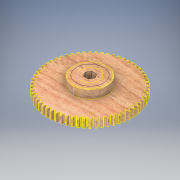
# Autodesk Inventor part: gear2
Saved by Autodesk Inventor 2018 (Build 220112000, 112)
## iProperties
Created: 2019-02-16
Part Number: gear2
Material: Generic
Description: SolidWorks IGES file using analytic representation for surfaces
Document SubType Name: Modeling
Designer: snipe
Density: 1 g/cm^3
Appearance: Default
Sending System: SolidWorks 2018
Preprocessor: SolidWorks 2018
Minimum Resolution: 0.0
Sending System Product ID: 48_gear2
Receiving System Product ID: 48_gear2
Sent Units: Millimeter
Translation Standard: IGES 5.3
Model Creation Time: 2019-02-16
Title: C:\Users\Admin\Desktop\48_gear2.IGS
Author: Admin
Autodesk Inventor part; units mm, degrees
ref_plane "YZ Plane" through (0, 0, 0) normal (1, 0, 0) x (0, 1, 0)
ref_plane "XZ Plane" through (0, 0, 0) normal (0, 1, 0) x (-1, 0, 0)
ref_plane "XY Plane" through (0, 0, 0) normal (0, 0, 1) x (1, 0, 0)
surface "Composite1"
sketch "Sketch1" plane through (0, 19, 0) normal (0, 1, 0) x (1, 0, 0)
  line L0 (7.3323, 0) -> (3.6662, -6.35)
  line L1 (3.6662, -6.35) -> (-3.6662, -6.35)
  line L2 (-3.6662, -6.35) -> (-7.3323, 0)
  line L3 (-7.3323, 0) -> (-3.6662, 6.35)
  line L4 (-3.6662, 6.35) -> (3.6662, 6.35)
  line L5 (3.6662, 6.35) -> (7.3323, 0)
  circle A0 centre (0, 0) radius 20
  dimension "d1" = 40
  dimension "d4" = 12.7
  constraints: 12 end point, 2 coincident, 1 centre point, 13 other
  measures "d1" diameter of A0
  measures "d4" distance between parallel lines of L1 L4
extrude "Extrusion1" add sketch "Sketch1" against normal up to surface (38 mm away)
body "Solid1"
body "Srf1"
